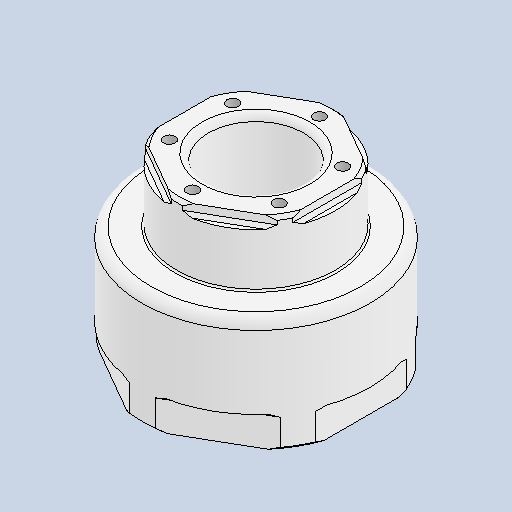
# Autodesk Inventor part: joint3_asix4
Saved by Autodesk Inventor 2025.3 (Build 293356030, 356C)
## iProperties
Created: 2025-11-24
Part Number: joint3_asix4
Material: PLA filament
Document SubType Name: Modeling
Designer: MSI
Mass: 168.889 g
Surface Area: 242.85 cm^2
Volume: 140.741 cm^3
Density: 1.2 g/cm^3
Appearance: 일반
Author: MSI
Autodesk Inventor part; units mm, degrees
ref_plane "YZ Plane" through (0, 0, 0) normal (1, 0, 0) x (0, 1, 0)
ref_plane "XZ Plane" through (0, 0, 0) normal (0, 1, 0) x (-1, 0, 0)
ref_plane "XY Plane" through (0, 0, 0) normal (0, 0, 1) x (1, 0, 0)
sketch "스케치1" plane through (0, 0, 0) normal (0, 0, 1) x (1, 0, 0)
  line L0 (0, 0) -> (36, 0)
  line L1 (36, 0) -> (36, 36.206)
  line L2 (36, 36.206) -> (0, 36.206)
  line L3 (0, 36.206) -> (0, 0)
  line L4 (0, 36.206) -> (25, 36.206)
  line L5 (25, 36.206) -> (25, 56.206)
  line L6 (25, 56.206) -> (0, 56.206)
  line L7 (0, 56.206) -> (0, 36.206)
  dimension "d0" = 50
  dimension "d1" = 72
  dimension "d2" = 36.206
  dimension "d3" = 56.206
  constraints: 16 end point, 4 parallel, 2 horizontal, 2 perpendicular
  measures "d0" diameter of L5 L7
  measures "d1" diameter of L1 L3
  measures "d2" distance of L0.end L1.end
  measures "d3" distance between parallel lines of L0 L6
revolve "회전1" add sketch "스케치1" angle 360 about axis through (0, 36.206, 0) along (0, -1, 0)
chamfer "모따기1" distance 1 angle 45 2 edges at (-36, 0, 0) (-25, 56.206, 0)
sketch "스케치2" plane through (0, 0, 0) normal (0, -1, 0) x (1, 0, 0)
  line L0 (0, -38.1051) -> (-33, -19.0526)
  line L1 (-33, -19.0526) -> (-33, 19.0526)
  line L2 (-33, 19.0526) -> (0, 38.1051)
  line L3 (0, 38.1051) -> (33, 19.0526)
  line L4 (33, 19.0526) -> (33, -19.0526)
  line L5 (33, -19.0526) -> (0, -38.1051)
  circle A0 centre (0, 0) radius 36 projected
  point P0 (0, 0)
  point P1 (0, 0)
  point P2 (4.0401, -35.7726)
  point P3 (28.9599, -21.3851)
  point P4 (-28.9599, -21.3851)
  point P5 (-4.0401, -35.7726)
  point P6 (33, 14.3875)
  point P7 (33, -14.3875)
  point P8 (-33, 14.3875)
  point P9 (-33, -14.3875)
  point P10 (28.9599, 21.3851)
  point P11 (4.0401, 35.7726)
  point P12 (-4.0401, 35.7726)
  point P13 (-28.9599, 21.3851)
  dimension "d5" = 66
  constraints: 12 end point, 1 coincident, 1 vertical, 13 other
  measures "d5" distance between parallel lines of L1 L4
extrude "돌출1" cut sketch "스케치2" against normal blind 10.25 contours L0 A0 L5 | A0 L0 | L5 A0 | L0 L1 A0 | A0 L4 L5 | A0 L1 | L4 A0 | L1 L2 A0 | A0 L3 L4 | A0 L2 | L3 A0 | L2 L3 A0
sketch "스케치3" plane through (0, 56.206, 0) normal (0, 1, 0) x (1, 0, 0)
  line L0 (0, 25.9808) -> (22.5, 12.9904)
  line L1 (22.5, 12.9904) -> (22.5, -12.9904)
  line L2 (22.5, -12.9904) -> (0, -25.9808)
  line L3 (0, -25.9808) -> (-22.5, -12.9904)
  line L4 (-22.5, -12.9904) -> (-22.5, 12.9904)
  line L5 (-22.5, 12.9904) -> (0, 25.9808)
  circle A0 centre (0, 0) radius 25 projected
  point P0 (0, 0)
  point P1 (1.8127, -24.9342)
  point P2 (20.6873, -14.0369)
  point P3 (-20.6873, -14.0369)
  point P4 (-1.8127, -24.9342)
  point P5 (22.5, 10.8972)
  point P6 (22.5, -10.8972)
  point P7 (-22.5, 10.8972)
  point P8 (-22.5, -10.8972)
  point P9 (20.6873, 14.0369)
  point P10 (1.8127, 24.9342)
  point P11 (-1.8127, 24.9342)
  point P12 (-20.6873, 14.0369)
  dimension "d8" = 45
  constraints: 12 end point, 1 coincident, 1 vertical, 13 other
  measures "d8" distance between parallel lines of L1 L4
extrude "돌출2" cut sketch "스케치3" against normal blind 3.25 contours L0 A0 L5 | A0 L0 | L5 A0 | L0 L1 A0 | A0 L4 L5 | A0 L1 | L4 A0 | L1 L2 A0 | A0 L3 L4 | A0 L2 | L3 A0 | L2 L3 A0
sketch "스케치6" plane through (0, 56.206, 0) normal (0, 1, 0) x (1, 0, 0)
  circle A0 centre (0, 0) radius 36 projected
  point P0 (0, 0)
  constraints: 1 coincident
hole "구멍3" at (0, 56.206, 0) direction (0, -1, 0) diameter 30 end through all
sketch "스케치4" plane through (0, 0, 0) normal (0, -1, 0) x (-0.5, 0, -0.8660254)
  line L0 (0, 0) -> (0, 24)
  dimension "d11" = 24
  constraints: 2 end point, 1 vertical
  measures "d11" distance of L0.start L0.end
hole "구멍1" at (20.7846, 0, -12) direction (0, 1, 0) diameter 3.6881 depth 13 tip angle 118 thread size "M4.5x0.75" class "6H" standard "ISO Metric profile"
sketch "스케치5" plane through (0, 56.206, 0) normal (0, 1, 0) x (-0.5, 0, 0.8660254)
  line L0 (0, 0) -> (0, -20)
  dimension "d19" = 20
  constraints: 2 end point, 1 vertical
  measures "d19" distance of L0.start L0.end
hole "구멍2" at (-17.3205, 56.206, -10) direction (0, -1, 0) diameter 3.6881 depth 10 tip angle 118 thread size "M4.5x0.75" class "6H" standard "ISO Metric profile"
pattern_circular "원형 패턴1" count 6 over 360 about axis through (0, 18.103, 0) along (0, -1, 0) of "구멍2", "구멍1"
chamfer "모따기2" distance 1 angle 45 12 edges at (16.5, 10.25, -28.5788) (-16.5, 10.25, -28.5788) (-33, 10.25, 0) (-16.5, 10.25, 28.5788) (16.5, 10.25, 28.5788) (33, 10.25, 0) (11.25, 52.956, -19.4856) (22.5, 52.956, 0) (11.25, 52.956, 19.4856) (-11.25, 52.956, 19.4856) (-22.5, 52.956, 0) (-11.25, 52.956, -19.4856)
fillet "모깎기1" radius 2 1 edges at (0, 56.206, -15)
fillet "모깎기2" radius 3 1 edges at (-36, 36.206, 0)
fillet "모깎기3" radius 0.5 1 edges at (-25, 36.206, 0)
equation "\"d0\" = joint3_axis4_d2"
equation "\"d36\" = joint3_axis4_d1"
equation "\"joint4_belt_centor\" = 157.367"
equation "\"joint4_axis2_L\" = 58.803"
equation "\"joint4_axis2_b1\" = 35"
equation "\"joint4_axis2_d\" = 19"
equation "\"joint4_miter_m\" = 2"
equation "\"joint4_miter_a\" = 20deg"
equation "\"joint4_miter_z\" = 79"
equation "\"joint4_miter_b\" = 6.90139"
equation "\"joint4_axis3_L\" = 23.5"
equation "\"joint3_belt_centor\" = 157.367"
equation "\"joint3_axis2_L\" = 63.75"
equation "\"joint3_axis2_b1\" = 38"
equation "\"joint3_axis2_d\" = 29"
equation "\"joint3_planetary_m\" = 2"
equation "\"joint3_planetary_a\" = 20deg"
equation "\"joint3_planetary_np\" = 4"
equation "\"joint3_sun_b\" = 19"
equation "\"joint3_planet_b\" = 19"
equation "\"joint3_ring_b\" = 18"
equation "\"joint3_axis3_d\" = 29"
equation "\"joint3_miter_m\" = 4"
equation "\"joint3_miter_a\" = 20deg"
equation "\"joint3_miter_z1\" = 26"
equation "\"joint3_miter_z2\" = 39"
equation "\"joint3_miter_b\" = 25.07657"
equation "\"joint3_axis4_L\" = 43.706"
equation "\"joint3_axis4_d1\" = 30"
equation "\"joint3_axis4_d2\" = 50"
